Autodesk Inventor part; units mm, degrees
(part 2 of 2)
  spline S7 degree 4 poles (70.4606, -93.4832) (71.6637, -94.3855) (72.0679, -94.9119) (72.6036, -95.4852) (72.6036, -95.6078) (73.7014, -97.389) (73.7885, -97.389) (73.7416, -97.2147) (72.716, -95.2037) (72.0591, -94.1982) (71.9853, -94.1513) (71.563, -93.9636) (70.4606, -93.4832) knots 1 1 1 1 1 2 3 4 5 6 7 8 9 10 10 10 10 10
  line L499 (62.8481, -98.9393) -> (62.8481, -106.5578)
  line L500 (62.8481, -98.9393) -> (62.8481, -99.488)
  line L501 (49.2759, -101.6069) -> (50.7433, -100.8509) construction
  line L502 (50.7433, -100.8509) -> (51.7824, -100.4569) construction
  line L503 (51.7824, -100.4569) -> (52.9356, -100.096) construction
  line L504 (52.9356, -100.096) -> (54.0835, -99.7847) construction
  line L505 (54.0835, -99.7847) -> (55.2643, -99.5619) construction
  line L506 (55.2643, -99.5619) -> (57.8656, -99.2086) construction
  line L507 (57.8656, -99.2086) -> (59.3023, -99.058) construction
  line L508 (59.3023, -99.058) -> (60.6779, -98.9782) construction
  line L509 (60.6779, -98.9782) -> (62.1962, -98.9393) construction
  line L510 (62.1962, -98.9393) -> (62.8481, -98.9393) construction
  spline S8 degree 4 poles (49.2759, -101.6069) (50.7433, -100.8509) (51.7824, -100.4569) (52.9356, -100.096) (54.0835, -99.7847) (55.2643, -99.5619) (57.8656, -99.2086) (59.3023, -99.058) (60.6779, -98.9782) (62.1962, -98.9393) (62.8481, -98.9393) knots 1 1 1 1 1 2 3 4 5 6 7 8 8 8 8 8
  line L511 (62.8481, -99.488) -> (61.3216, -99.488) construction
  line L512 (61.3216, -99.488) -> (60.1322, -99.5392) construction
  line L513 (60.1322, -99.5392) -> (58.753, -99.6193) construction
  line L514 (58.753, -99.6193) -> (56.3595, -99.8521) construction
  line L515 (56.3595, -99.8521) -> (54.7558, -100.1468) construction
  line L516 (54.7558, -100.1468) -> (53.0368, -100.4342) construction
  line L517 (53.0368, -100.4342) -> (51.7707, -100.7521) construction
  line L518 (51.7707, -100.7521) -> (50.7899, -101.0685) construction
  line L519 (50.7899, -101.0685) -> (50.2272, -101.2734) construction
  line L520 (50.2272, -101.2734) -> (49.8128, -101.4306) construction
  line L521 (49.8128, -101.4306) -> (49.3786, -101.568) construction
  line L522 (49.3786, -101.568) -> (49.2759, -101.6069) construction
  spline S9 degree 4 poles (62.8481, -99.488) (61.3216, -99.488) (60.1322, -99.5392) (58.753, -99.6193) (56.3595, -99.8521) (54.7558, -100.1468) (53.0368, -100.4342) (51.7707, -100.7521) (50.7899, -101.0685) (50.2272, -101.2734) (49.8128, -101.4306) (49.3786, -101.568) (49.2759, -101.6069) knots 1 1 1 1 1 2 3 4 5 6 7 8 9 10 10 10 10 10
  line L523 (54.5141, -102.0673) -> (55.0222, -101.6163) construction
  line L524 (55.0222, -101.6163) -> (55.3711, -101.3631) construction
  line L525 (55.3711, -101.3631) -> (55.7133, -101.171) construction
  line L526 (55.7133, -101.171) -> (56.2006, -100.9503) construction
  line L527 (56.2006, -100.9503) -> (56.8732, -100.6623) construction
  line L528 (56.8732, -100.6623) -> (57.4218, -100.4315) construction
  line L529 (57.4218, -100.4315) -> (57.9242, -100.2486) construction
  line L530 (57.9242, -100.2486) -> (58.2333, -100.1355) construction
  line L531 (58.2333, -100.1355) -> (58.9999, -99.8891) construction
  line L532 (58.9999, -99.8891) -> (59.3785, -99.7778) construction
  line L533 (59.3785, -99.7778) -> (59.5633, -99.7307) construction
  spline S10 degree 4 poles (54.5141, -102.0673) (55.0222, -101.6163) (55.3711, -101.3631) (55.7133, -101.171) (56.2006, -100.9503) (56.8732, -100.6623) (57.4218, -100.4315) (57.9242, -100.2486) (58.2333, -100.1355) (58.9999, -99.8891) (59.3785, -99.7778) (59.5633, -99.7307) knots 1 1 1 1 1 2 3 4 5 6 7 8 9 9 9 9 9
  line L534 (59.5633, -99.7307) -> (58.9599, -100.035) construction
  line L535 (58.9599, -100.035) -> (58.6826, -100.171) construction
  line L536 (58.6826, -100.171) -> (58.3642, -100.3143) construction
  line L537 (58.3642, -100.3143) -> (57.9551, -100.5268) construction
  line L538 (57.9551, -100.5268) -> (57.6463, -100.6623) construction
  line L539 (57.6463, -100.6623) -> (57.2926, -100.8458) construction
  line L540 (57.2926, -100.8458) -> (56.6189, -101.1343) construction
  line L541 (56.6189, -101.1343) -> (55.9395, -101.4897) construction
  line L542 (55.9395, -101.4897) -> (54.5141, -102.0673) construction
  spline S11 degree 4 poles (59.5633, -99.7307) (58.9599, -100.035) (58.6826, -100.171) (58.3642, -100.3143) (57.9551, -100.5268) (57.6463, -100.6623) (57.2926, -100.8458) (56.6189, -101.1343) (55.9395, -101.4897) (54.5141, -102.0673) knots 1 1 1 1 1 2 3 4 5 6 7 7 7 7 7
  line L543 (58.8578, -103.276) -> (58.913, -103.1477) construction
  line L544 (60.1013, -101.7124) -> (60.3468, -101.4787) construction
  line L545 (60.3468, -101.4787) -> (60.872, -101.0319) construction
  line L546 (60.872, -101.0319) -> (61.2903, -100.6758) construction
  line L547 (61.2903, -100.6758) -> (61.7041, -100.3756) construction
  line L548 (61.7041, -100.3756) -> (61.9485, -100.1984) construction
  line L549 (61.9485, -100.1984) -> (62.295, -99.9994) construction
  spline S12 degree 4 poles (58.8578, -103.276) (58.913, -103.1477) (58.9946, -103.0128) (59.1388, -102.7938) (59.4687, -102.3614) (59.7813, -102.0376) (60.1013, -101.7124) (60.3468, -101.4787) (60.872, -101.0319) (61.2903, -100.6758) (61.7041, -100.3756) (61.9485, -100.1984) (62.295, -99.9994) knots 1 1 1 1 1 1.158039 1.166811 1.450335 2 3 4 5 6 7 7 7 7 7
  line L550 (58.8578, -103.276) -> (59.4042, -102.7553) construction
  line L551 (59.4042, -102.7553) -> (60.0215, -102.1676) construction
  line L552 (60.0215, -102.1676) -> (60.5755, -101.5874) construction
  line L553 (60.5755, -101.5874) -> (61.1809, -101.0444) construction
  line L554 (61.1809, -101.0444) -> (61.4836, -100.7761) construction
  line L555 (61.4836, -100.7761) -> (61.863, -100.4128) construction
  line L556 (61.863, -100.4128) -> (62.295, -99.9994) construction
  spline S13 degree 4 poles (58.8578, -103.276) (59.4042, -102.7553) (60.0215, -102.1676) (60.5755, -101.5874) (61.1809, -101.0444) (61.4836, -100.7761) (61.863, -100.4128) (62.295, -99.9994) knots 1 1 1 1 1 2 3 4 5 5 5 5 5
  line L557 (58.913, -103.1477) -> (58.9946, -103.0128) construction
  line L558 (59.7813, -102.0376) -> (60.1013, -101.7124) construction
  line L559 (58.9946, -103.0128) -> (59.1388, -102.7938) construction
  line L560 (59.1388, -102.7938) -> (59.4687, -102.3614) construction
  line L561 (59.4687, -102.3614) -> (59.7813, -102.0376) construction
  line L562 (62.8481, -101.1343) -> (61.5548, -101.1343) construction
  line L563 (61.5548, -101.1343) -> (61.1724, -101.1214) construction
  line L564 (61.1724, -101.1214) -> (60.4661, -101.0924) construction
  line L565 (60.4661, -101.0924) -> (59.0371, -100.9585) construction
  line L566 (59.0371, -100.9585) -> (57.4305, -100.8064) construction
  line L567 (57.4305, -100.8064) -> (56.0608, -100.6236) construction
  line L568 (56.0608, -100.6236) -> (54.5965, -100.3756) construction
  line L569 (54.5965, -100.3756) -> (53.7703, -100.2061) construction
  spline S14 degree 4 poles (62.8481, -101.1343) (61.5548, -101.1343) (61.1724, -101.1214) (60.4661, -101.0924) (59.0371, -100.9585) (57.4305, -100.8064) (56.0608, -100.6236) (54.5965, -100.3756) (53.7703, -100.2061) knots 1 1 1 1 1 2 3 4 5 6 6 6 6 6
  line L570 (53.7703, -100.2061) -> (53.7454, -100.2765) construction
  line L571 (53.7454, -100.2765) -> (53.7995, -100.2765) construction
  line L572 (53.7995, -100.2765) -> (53.9785, -100.3525) construction
  line L573 (53.9785, -100.3525) -> (54.4473, -100.4901) construction
  line L574 (54.4473, -100.4901) -> (54.8747, -100.6058) construction
  line L575 (54.8747, -100.6058) -> (55.6292, -100.754) construction
  line L576 (55.6292, -100.754) -> (56.0992, -100.8349) construction
  line L577 (56.0992, -100.8349) -> (56.4446, -100.8935) construction
  line L578 (56.4446, -100.8935) -> (57.4616, -101.0606) construction
  line L579 (57.4616, -101.0606) -> (58.7366, -101.2012) construction
  line L580 (58.7366, -101.2012) -> (59.815, -101.2852) construction
  line L581 (59.815, -101.2852) -> (60.4661, -101.3281) construction
  line L582 (60.4661, -101.3281) -> (61.3133, -101.3631) construction
  line L583 (61.3133, -101.3631) -> (62.2784, -101.3852) construction
  line L584 (62.2784, -101.3852) -> (62.8481, -101.3852) construction
  spline S15 degree 4 poles (53.7703, -100.2061) (53.7454, -100.2765) (53.7995, -100.2765) (53.9785, -100.3525) (54.4473, -100.4901) (54.8747, -100.6058) (55.6292, -100.754) (56.0992, -100.8349) (56.4446, -100.8935) (57.4616, -101.0606) (58.7366, -101.2012) (59.815, -101.2852) (60.4661, -101.3281) (61.3133, -101.3631) (62.2784, -101.3852) (62.8481, -101.3852) knots 1 1 1 1 1 2 3 4 5 6 7 8 9 10 11 12 13 13 13 13 13
  line L585 (62.8481, -101.1343) -> (62.8481, -101.3852)
  line L586 (76.4202, -101.6069) -> (74.9528, -100.8509) construction
  line L587 (74.9528, -100.8509) -> (73.9137, -100.4569) construction
  line L588 (73.9137, -100.4569) -> (72.7605, -100.096) construction
  line L589 (72.7605, -100.096) -> (71.6126, -99.7847) construction
  line L590 (71.6126, -99.7847) -> (70.4318, -99.5619) construction
  line L591 (70.4318, -99.5619) -> (67.8305, -99.2086) construction
  line L592 (67.8305, -99.2086) -> (66.3938, -99.058) construction
  line L593 (66.3938, -99.058) -> (65.0182, -98.9782) construction
  line L594 (65.0182, -98.9782) -> (63.4999, -98.9393) construction
  line L595 (63.4999, -98.9393) -> (62.8481, -98.9393) construction
  spline S16 degree 4 poles (76.4202, -101.6069) (74.9528, -100.8509) (73.9137, -100.4569) (72.7605, -100.096) (71.6126, -99.7847) (70.4318, -99.5619) (67.8305, -99.2086) (66.3938, -99.058) (65.0182, -98.9782) (63.4999, -98.9393) (62.8481, -98.9393) knots 1 1 1 1 1 2 3 4 5 6 7 8 8 8 8 8
  line L596 (62.8481, -99.488) -> (64.3745, -99.488) construction
  line L597 (64.3745, -99.488) -> (65.564, -99.5392) construction
  line L598 (65.564, -99.5392) -> (66.9431, -99.6193) construction
  line L599 (66.9431, -99.6193) -> (69.3366, -99.8521) construction
  line L600 (69.3366, -99.8521) -> (70.9403, -100.1468) construction
  line L601 (70.9403, -100.1468) -> (72.6593, -100.4342) construction
  line L602 (72.6593, -100.4342) -> (73.9254, -100.7521) construction
  line L603 (73.9254, -100.7521) -> (74.9062, -101.0685) construction
  line L604 (74.9062, -101.0685) -> (75.469, -101.2734) construction
  line L605 (75.469, -101.2734) -> (75.8833, -101.4306) construction
  line L606 (75.8833, -101.4306) -> (76.3175, -101.568) construction
  line L607 (76.3175, -101.568) -> (76.4202, -101.6069) construction
  spline S17 degree 4 poles (62.8481, -99.488) (64.3745, -99.488) (65.564, -99.5392) (66.9431, -99.6193) (69.3366, -99.8521) (70.9403, -100.1468) (72.6593, -100.4342) (73.9254, -100.7521) (74.9062, -101.0685) (75.469, -101.2734) (75.8833, -101.4306) (76.3175, -101.568) (76.4202, -101.6069) knots 1 1 1 1 1 2 3 4 5 6 7 8 9 10 10 10 10 10
  line L608 (71.182, -102.0673) -> (70.6739, -101.6163) construction
  line L609 (70.6739, -101.6163) -> (70.325, -101.3631) construction
  line L610 (70.325, -101.3631) -> (69.9828, -101.171) construction
  line L611 (69.9828, -101.171) -> (69.4955, -100.9503) construction
  line L612 (69.4955, -100.9503) -> (68.8229, -100.6623) construction
  line L613 (68.8229, -100.6623) -> (68.2743, -100.4315) construction
  line L614 (68.2743, -100.4315) -> (67.7719, -100.2486) construction
  line L615 (67.7719, -100.2486) -> (67.4628, -100.1355) construction
  line L616 (67.4628, -100.1355) -> (66.6962, -99.8891) construction
  line L617 (66.6962, -99.8891) -> (66.3176, -99.7778) construction
  line L618 (66.3176, -99.7778) -> (66.1328, -99.7307) construction
  spline S18 degree 4 poles (71.182, -102.0673) (70.6739, -101.6163) (70.325, -101.3631) (69.9828, -101.171) (69.4955, -100.9503) (68.8229, -100.6623) (68.2743, -100.4315) (67.7719, -100.2486) (67.4628, -100.1355) (66.6962, -99.8891) (66.3176, -99.7778) (66.1328, -99.7307) knots 1 1 1 1 1 2 3 4 5 6 7 8 9 9 9 9 9
  line L619 (66.1328, -99.7307) -> (66.7363, -100.035) construction
  line L620 (66.7363, -100.035) -> (67.0135, -100.171) construction
  line L621 (67.0135, -100.171) -> (67.3319, -100.3143) construction
  line L622 (67.3319, -100.3143) -> (67.741, -100.5268) construction
  line L623 (67.741, -100.5268) -> (68.0498, -100.6623) construction
  line L624 (68.0498, -100.6623) -> (68.4035, -100.8458) construction
  line L625 (68.4035, -100.8458) -> (69.0772, -101.1343) construction
  line L626 (69.0772, -101.1343) -> (69.7566, -101.4897) construction
  line L627 (69.7566, -101.4897) -> (71.182, -102.0673) construction
  spline S19 degree 4 poles (66.1328, -99.7307) (66.7363, -100.035) (67.0135, -100.171) (67.3319, -100.3143) (67.741, -100.5268) (68.0498, -100.6623) (68.4035, -100.8458) (69.0772, -101.1343) (69.7566, -101.4897) (71.182, -102.0673) knots 1 1 1 1 1 2 3 4 5 6 7 7 7 7 7
  line L628 (66.8383, -103.276) -> (66.7831, -103.1477) construction
  line L629 (65.5948, -101.7124) -> (65.3493, -101.4787) construction
  line L630 (65.3493, -101.4787) -> (64.8241, -101.0319) construction
  line L631 (64.8241, -101.0319) -> (64.4058, -100.6758) construction
  line L632 (64.4058, -100.6758) -> (63.992, -100.3756) construction
  line L633 (63.992, -100.3756) -> (63.7476, -100.1984) construction
  line L634 (63.7476, -100.1984) -> (63.4011, -99.9994) construction
  spline S20 degree 4 poles (66.8383, -103.276) (66.7831, -103.1477) (66.7015, -103.0128) (66.5573, -102.7938) (66.2274, -102.3614) (65.9148, -102.0376) (65.5948, -101.7124) (65.3493, -101.4787) (64.8241, -101.0319) (64.4058, -100.6758) (63.992, -100.3756) (63.7476, -100.1984) (63.4011, -99.9994) knots 1 1 1 1 1 1.158039 1.166811 1.450335 2 3 4 5 6 7 7 7 7 7
  line L635 (66.8383, -103.276) -> (66.2919, -102.7553) construction
  line L636 (66.2919, -102.7553) -> (65.6746, -102.1676) construction
  line L637 (65.6746, -102.1676) -> (65.1207, -101.5874) construction
  line L638 (65.1207, -101.5874) -> (64.5152, -101.0444) construction
  line L639 (64.5152, -101.0444) -> (64.2125, -100.7761) construction
  line L640 (64.2125, -100.7761) -> (63.8331, -100.4128) construction
  line L641 (63.8331, -100.4128) -> (63.4011, -99.9994) construction
  spline S21 degree 4 poles (66.8383, -103.276) (66.2919, -102.7553) (65.6746, -102.1676) (65.1207, -101.5874) (64.5152, -101.0444) (64.2125, -100.7761) (63.8331, -100.4128) (63.4011, -99.9994) knots 1 1 1 1 1 2 3 4 5 5 5 5 5
  line L642 (66.7831, -103.1477) -> (66.7015, -103.0128) construction
  line L643 (65.9148, -102.0376) -> (65.5948, -101.7124) construction
  line L644 (66.7015, -103.0128) -> (66.5573, -102.7938) construction
  line L645 (66.5573, -102.7938) -> (66.2274, -102.3614) construction
  line L646 (66.2274, -102.3614) -> (65.9148, -102.0376) construction
  line L647 (62.8481, -101.1343) -> (64.1413, -101.1343) construction
  line L648 (64.1413, -101.1343) -> (64.5237, -101.1214) construction
  line L649 (64.5237, -101.1214) -> (65.23, -101.0924) construction
  line L650 (65.23, -101.0924) -> (66.659, -100.9585) construction
  line L651 (66.659, -100.9585) -> (68.2656, -100.8064) construction
  line L652 (68.2656, -100.8064) -> (69.6353, -100.6236) construction
  line L653 (69.6353, -100.6236) -> (71.0996, -100.3756) construction
  line L654 (71.0996, -100.3756) -> (71.9258, -100.2061) construction
  spline S22 degree 4 poles (62.8481, -101.1343) (64.1413, -101.1343) (64.5237, -101.1214) (65.23, -101.0924) (66.659, -100.9585) (68.2656, -100.8064) (69.6353, -100.6236) (71.0996, -100.3756) (71.9258, -100.2061) knots 1 1 1 1 1 2 3 4 5 6 6 6 6 6
  line L655 (71.9258, -100.2061) -> (71.9507, -100.2765) construction
  line L656 (71.9507, -100.2765) -> (71.8966, -100.2765) construction
  line L657 (71.8966, -100.2765) -> (71.7176, -100.3525) construction
  line L658 (71.7176, -100.3525) -> (71.2488, -100.4901) construction
  line L659 (71.2488, -100.4901) -> (70.8215, -100.6058) construction
  line L660 (70.8215, -100.6058) -> (70.0669, -100.754) construction
  line L661 (70.0669, -100.754) -> (69.597, -100.8349) construction
  line L662 (69.597, -100.8349) -> (69.2515, -100.8935) construction
  line L663 (69.2515, -100.8935) -> (68.2345, -101.0606) construction
  line L664 (68.2345, -101.0606) -> (66.9595, -101.2012) construction
  line L665 (66.9595, -101.2012) -> (65.8811, -101.2852) construction
  line L666 (65.8811, -101.2852) -> (65.23, -101.3281) construction
  line L667 (65.23, -101.3281) -> (64.3828, -101.3631) construction
  line L668 (64.3828, -101.3631) -> (63.4177, -101.3852) construction
  line L669 (63.4177, -101.3852) -> (62.8481, -101.3852) construction
  spline S23 degree 4 poles (71.9258, -100.2061) (71.9507, -100.2765) (71.8966, -100.2765) (71.7176, -100.3525) (71.2488, -100.4901) (70.8215, -100.6058) (70.0669, -100.754) (69.597, -100.8349) (69.2515, -100.8935) (68.2345, -101.0606) (66.9595, -101.2012) (65.8811, -101.2852) (65.23, -101.3281) (64.3828, -101.3631) (63.4177, -101.3852) (62.8481, -101.3852) knots 1 1 1 1 1 2 3 4 5 6 7 8 9 10 11 12 13 13 13 13 13
  point P0 (0, 0)
  constraints: 82 symmetric about line, 27 perpendicular, 22 parallel, 21 horizontal, 10 vertical, 6 end point, 3 point on line, 1 collinear, 64 other
extrude "Выдавливание5" add sketch "Эскиз6" along normal blind 0.1 contours S0 | S16 S17 S23 S22 L499 | L499 S9 S14 S15 S8 | S22 S21 S23 L499 | L499 S15 S13 S14 | S14 S10 S15 S9 | S9 S15 S14 | S22 S23 S17 | S17 S23 S18 S22 | S14 S12 S13 | S13 S15 S12 S14 | S22 S20 S23 S21 | S21 S20 S22 | S14 S11 S15 S10 | S10 S11 S14 | S22 S19 S18 | S18 S23 S19 S22 | S15 S11 S10 | S18 S19 S23 | S13 S12 S15 | S23 S20 S21 | S12 S15 S11 S14 | S22 S19 S23 S20
sketch "Эскиз7" plane through (0, 0, 4) normal (0, 0, 1) x (1, 0, 0)
  line L0 (77.3024, -92.2561) -> (130.1224, -92.2561) construction
  line L1 (130.1224, -92.2561) -> (130.1224, -98.6605) construction
  line L2 (130.1224, -98.6605) -> (77.3024, -98.6605) construction
  line L3 (77.3024, -98.6605) -> (77.3024, -92.2561) construction
  line L4 (77.8221, -92.3427) -> (81.6383, -92.3427)
  line L5 (81.6383, -92.3427) -> (81.6383, -93.4159)
  line L6 (81.6383, -93.4159) -> (79.3765, -93.4159)
  line L7 (79.3765, -93.4159) -> (79.3765, -94.2869)
  line L8 (79.3765, -94.2869) -> (81.3062, -94.2869)
  line L9 (81.3062, -94.2869) -> (81.3062, -95.2975)
  line L10 (81.3062, -95.2975) -> (79.3765, -95.2975)
  line L11 (79.3765, -95.2975) -> (79.3765, -97.3427)
  line L12 (79.3765, -97.3427) -> (77.8221, -97.3427)
  line L13 (77.8221, -97.3427) -> (77.8221, -92.3427)
  line L14 (82.4756, -92.3427) -> (84.0204, -92.3427)
  line L15 (84.0204, -92.3427) -> (84.0204, -96.1108)
  line L16 (84.0204, -96.1108) -> (86.4314, -96.1108)
  line L17 (86.4314, -96.1108) -> (86.4314, -97.3427)
  line L18 (86.4314, -97.3427) -> (82.4756, -97.3427)
  line L19 (82.4756, -97.3427) -> (82.4756, -92.3427)
  line L20 (86.6335, -92.3427) -> (88.3515, -92.3427)
  line L21 (88.3515, -92.3427) -> (89.3572, -94.0271)
  line L22 (89.3572, -94.0271) -> (90.3678, -92.3427)
  line L23 (90.3678, -92.3427) -> (92.0762, -92.3427)
  line L24 (92.0762, -92.3427) -> (90.132, -95.2494)
  line L25 (90.132, -95.2494) -> (90.132, -97.3427)
  line L26 (90.132, -97.3427) -> (88.5825, -97.3427)
  line L27 (88.5825, -97.3427) -> (88.5825, -95.2494)
  line L28 (88.5825, -95.2494) -> (86.6335, -92.3427)
  line L29 (92.6392, -92.3427) -> (94.1888, -92.3427)
  line L30 (94.1888, -92.3427) -> (94.1888, -97.3427)
  line L31 (94.1888, -97.3427) -> (92.6392, -97.3427)
  line L32 (92.6392, -97.3427) -> (92.6392, -92.3427)
  line L33 (95.3053, -92.3427) -> (96.749, -92.3427)
  line L34 (96.749, -92.3427) -> (98.6354, -95.1098)
  line L35 (98.6354, -95.1098) -> (98.6354, -92.3427)
  line L36 (98.6354, -92.3427) -> (100.0935, -92.3427)
  line L37 (100.0935, -92.3427) -> (100.0935, -97.3427)
  line L38 (100.0935, -97.3427) -> (98.6354, -97.3427)
  line L39 (98.6354, -97.3427) -> (96.7586, -94.5901)
  line L40 (96.7586, -94.5901) -> (96.7586, -97.3427)
  line L41 (96.7586, -97.3427) -> (95.3053, -97.3427)
  line L42 (95.3053, -97.3427) -> (95.3053, -92.3427)
  line L43 (103.6402, -95.5333) -> (103.6402, -94.4939)
  line L44 (103.6402, -94.4939) -> (106.0271, -94.4939)
  line L45 (106.0271, -94.4939) -> (106.0271, -96.6209)
  spline S0 degree 2 poles (106.0271, -96.6209) (105.339, -97.0925) (104.2851, -97.4294) (103.5632, -97.4294) knots 0 0 0 1 2 2 2
  spline S1 degree 2 poles (103.5632, -97.4294) (102.6729, -97.4294) (101.5468, -96.823) (100.9309, -95.6199) (100.9309, -94.8403) knots 0 0 0 1 2 3 3 3
  spline S2 degree 2 poles (100.9309, -94.8403) (100.9309, -94.0222) (101.6046, -92.8144) (102.2591, -92.4967) knots 0 0 0 1 2 2 2
  spline S3 degree 2 poles (102.2591, -92.4967) (102.7692, -92.2561) (103.6258, -92.2561) knots 0 0 0 1 1 1
  spline S4 degree 2 poles (103.6258, -92.2561) (104.4583, -92.2561) (105.2812, -92.5545) (105.825, -93.1897) (105.9597, -93.6709) knots 0 0 0 1 2 3 3 3
  line L46 (105.9597, -93.6709) -> (104.4679, -93.9404)
  spline S5 degree 2 poles (104.4679, -93.9404) (104.3765, -93.6565) (103.9338, -93.3533) (103.5921, -93.3533) knots 0 0 0 1 2 2 2
  spline S6 degree 2 poles (103.5921, -93.3533) (103.0868, -93.3533) (102.4804, -94.0607) (102.4804, -94.8259) knots 0 0 0 1 2 2 2
  spline S7 degree 2 poles (102.4804, -94.8259) (102.4804, -95.6344) (103.0916, -96.3322) (103.6402, -96.3322) knots 0 0 0 1 2 2 2
  spline S8 degree 2 poles (103.6402, -96.3322) (103.9001, -96.3322) (104.3717, -96.183) (104.6749, -96.0001) knots 0 0 0 1 2 2 2
  line L47 (104.6749, -96.0001) -> (104.6749, -95.5333)
  line L48 (104.6749, -95.5333) -> (103.6402, -95.5333)
  line L49 (109.2754, -92.3427) -> (112.1676, -92.3427)
  spline S9 degree 2 poles (112.1676, -92.3427) (112.8895, -92.3427) (113.6643, -93.0598) (113.6643, -93.5891) knots 0 0 0 1 2 2 2
  spline S10 degree 2 poles (113.6643, -93.5891) (113.6643, -94.0319) (113.39, -94.3495) knots 0 0 0 1 1 1
  spline S11 degree 2 poles (113.39, -94.3495) (113.2023, -94.5612) (112.8462, -94.6863) knots 0 0 0 1 1 1
  spline S12 degree 2 poles (112.8462, -94.6863) (113.3852, -94.8163) (113.8953, -95.4467) (113.8953, -95.9231) knots 0 0 0 1 2 2 2
  spline S13 degree 2 poles (113.8953, -95.9231) (113.8953, -96.3081) (113.5343, -96.9289) (113.2215, -97.1118) knots 0 0 0 1 2 2 2
  spline S14 degree 2 poles (113.2215, -97.1118) (113.0242, -97.2224) (112.6344, -97.2754) knots 0 0 0 1 1 1
  spline S15 degree 2 poles (112.6344, -97.2754) (112.1099, -97.3427) (111.9415, -97.3427) knots 0 0 0 1 1 1
  line L50 (111.9415, -97.3427) -> (109.2754, -97.3427)
  line L51 (109.2754, -97.3427) -> (109.2754, -92.3427)
  line L52 (110.8346, -96.2696) -> (111.619, -96.2696)
  spline S16 degree 2 poles (111.619, -96.2696) (112.0185, -96.2696) (112.3457, -95.9857) (112.3457, -95.7499) knots 0 0 0 1 2 2 2
  spline S17 degree 2 poles (112.3457, -95.7499) (112.3457, -95.5285) (112.0233, -95.259) (111.619, -95.259) knots 0 0 0 1 2 2 2
  line L53 (111.619, -95.259) -> (110.8346, -95.259)
  line L54 (110.8346, -95.259) -> (110.8346, -96.2696)
  line L55 (110.8346, -94.3062) -> (111.5035, -94.3062)
  spline S18 degree 2 poles (111.5035, -94.3062) (111.8645, -94.3062) (112.1484, -94.0559) (112.1484, -93.8201) knots 0 0 0 1 2 2 2
  spline S19 degree 2 poles (112.1484, -93.8201) (112.1484, -93.6036) (111.8645, -93.3581) (111.5132, -93.3581) knots 0 0 0 1 2 2 2
  line L56 (111.5132, -93.3581) -> (110.8346, -93.3581)
  line L57 (110.8346, -93.3581) -> (110.8346, -94.3062)
  line L58 (114.7085, -92.3427) -> (118.8471, -92.3427)
  line L59 (118.8471, -92.3427) -> (118.8471, -93.4111)
  line L60 (118.8471, -93.4111) -> (116.2581, -93.4111)
  line L61 (116.2581, -93.4111) -> (116.2581, -94.2051)
  line L62 (116.2581, -94.2051) -> (118.6595, -94.2051)
  line L63 (118.6595, -94.2051) -> (118.6595, -95.2253)
  line L64 (118.6595, -95.2253) -> (116.2581, -95.2253)
  line L65 (116.2581, -95.2253) -> (116.2581, -96.2119)
  line L66 (116.2581, -96.2119) -> (118.9241, -96.2119)
  line L67 (118.9241, -96.2119) -> (118.9241, -97.3427)
  line L68 (118.9241, -97.3427) -> (114.7085, -97.3427)
  line L69 (114.7085, -97.3427) -> (114.7085, -92.3427)
  line L70 (122.8317, -96.515) -> (121.0752, -96.515)
  line L71 (121.0752, -96.515) -> (120.8298, -97.3427)
  line L72 (120.8298, -97.3427) -> (119.2514, -97.3427)
  line L73 (119.2514, -97.3427) -> (121.133, -92.3427)
  line L74 (121.133, -92.3427) -> (122.8221, -92.3427)
  line L75 (122.8221, -92.3427) -> (124.6989, -97.3427)
  line L76 (124.6989, -97.3427) -> (123.082, -97.3427)
  line L77 (123.082, -97.3427) -> (122.8317, -96.515)
  line L78 (122.5093, -95.4323) -> (121.9607, -93.6373)
  line L79 (121.9607, -93.6373) -> (121.4121, -95.4323)
  line L80 (121.4121, -95.4323) -> (122.5093, -95.4323)
  line L81 (125.2186, -97.3427) -> (125.2186, -92.3427)
  line L82 (125.2186, -92.3427) -> (127.7932, -92.3427)
  spline S20 degree 2 poles (127.7932, -92.3427) (128.5055, -92.3427) (129.2658, -92.5882) (129.7278, -93.2523) (129.7278, -93.7287) knots 0 0 0 1 2 3 3 3
  spline S21 degree 2 poles (129.7278, -93.7287) (129.7278, -94.1474) (129.3717, -94.7489) (129.0637, -94.9366) knots 0 0 0 1 2 2 2
  spline S22 degree 2 poles (129.0637, -94.9366) (128.8664, -95.0569) (128.5199, -95.1339) knots 0 0 0 1 1 1
  spline S23 degree 2 poles (128.5199, -95.1339) (128.7942, -95.2253) (128.9241, -95.3168) knots 0 0 0 1 1 1
  spline S24 degree 2 poles (128.9241, -95.3168) (129.0059, -95.3793) (129.3284, -95.7836) (129.3861, -95.8942) knots 0 0 0 1 2 2 2
  line L83 (129.3861, -95.8942) -> (130.132, -97.3427)
  line L84 (130.132, -97.3427) -> (128.3852, -97.3427)
  line L85 (128.3852, -97.3427) -> (127.5622, -95.8124)
  spline S25 degree 2 poles (127.5622, -95.8124) (127.4083, -95.5189) (127.2879, -95.4274) knots 0 0 0 1 1 1
  spline S26 degree 2 poles (127.2879, -95.4274) (127.1195, -95.3119) (126.9078, -95.3119) knots 0 0 0 1 1 1
  line L86 (126.9078, -95.3119) -> (126.773, -95.3119)
  line L87 (126.773, -95.3119) -> (126.773, -97.3427)
  line L88 (126.773, -97.3427) -> (125.2186, -97.3427)
  line L89 (126.773, -94.3687) -> (127.4227, -94.3687)
  spline S27 degree 2 poles (127.4227, -94.3687) (127.5238, -94.3687) (127.8269, -94.3014) knots 0 0 0 1 1 1
  spline S28 degree 2 poles (127.8269, -94.3014) (127.9809, -94.2677) (128.1734, -94.0174) (128.1734, -93.8538) knots 0 0 0 1 2 2 2
  spline S29 degree 2 poles (128.1734, -93.8538) (128.1734, -93.6132) (127.8702, -93.3533) (127.4468, -93.3533) knots 0 0 0 1 2 2 2
  line L90 (127.4468, -93.3533) -> (126.773, -93.3533)
  line L91 (126.773, -93.3533) -> (126.773, -94.3687)
  point P0 (0, 0)
  constraints: 2 other
extrude "Выдавливание6" add sketch "Эскиз7" along normal blind 0.1
